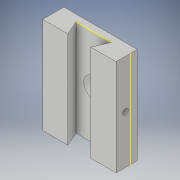
# Autodesk Inventor part: 7.1 Schlitten
Saved by Autodesk Inventor 2018.3 (Build 223284000, 284)
## iProperties
Created: 2018-10-11
Part Number: 7.1 Schlitten
Material: Generisch
Document SubType Name: Modeling
Designer: pgmadmin
Density: 1 g/cm^3
Appearance: Vorgabe
Author: pgmadmin
Autodesk Inventor part; units mm, degrees
ref_plane "YZ Plane" through (0, 0, 0) normal (1, 0, 0) x (0, 1, 0)
ref_plane "XZ Plane" through (0, 0, 0) normal (0, 1, 0) x (-1, 0, 0)
ref_plane "XY Plane" through (0, 0, 0) normal (0, 0, 1) x (1, 0, 0)
sketch "Skizze1" plane through (0, 0, 0) normal (0, 0, 1) x (1, 0, 0)
  line L0 (-18.1618, 0.375) -> (-21.3761, 7.875)
  line L1 (-2.9476, 7.875) -> (-6.1618, 0.375)
  line L2 (-6.1618, 0.375) -> (-18.1618, 0.375)
  line L3 (-18.1618, 0.375) -> (-31.1618, 0.375)
  line L4 (-31.1618, 0.375) -> (-31.1618, 11.375)
  line L5 (-31.1618, 11.375) -> (6.8382, 11.375)
  line L6 (6.8382, 11.375) -> (6.8382, 0.375)
  line L7 (6.8382, 0.375) -> (-6.1618, 0.375)
  line L8 (-21.5376, 7.875) -> (-2.9476, 7.875)
  point P0 (0, 0)
  point P1 (-21.1618, 7.375)
  point P2 (-3.1618, 7.375)
  dimension "d10" = 38
  dimension "d14" = 12
  dimension "d29" = 13
  constraints: 18 end point, 4 perpendicular, 4 point on line, 2 horizontal, 1 collinear
  measures "d10" distance of L4.end L5.end
  measures "d14" distance of L1.end L0.start
  measures "d29" distance of L0.start L3.end
extrude "Extrusion1" add sketch "Skizze1" along normal blind 50 contours L3 L4 L5 L6 L7 L1 L8 L0
sketch "Skizze2" plane through (6.8382, 0.375, 0) normal (1, 0, 0) x (0, 0, -1)
  line L0 (-50, 0) -> (-50, 11) projected
  line L1 (0, 11) -> (-50, 11) projected
  point P0 (0, -0.375)
  point P1 (-25, 4.85)
  dimension "d19" = 6.15
  measures "d19" distance from line of L1 point (-25, 4.85)
hole "Bohrung1" at (6.8382, 5.225, 25) direction (-1, 0, 0) diameter 2.9 depth 8 tip angle 118
sketch "Skizze3" plane through (-21.3761, 7.875, 0) normal (0, -1, 0) x (1, 0, 0)
  line L0 (0, 50) -> (18.4286, 50) projected
  line L1 (28.2143, 0) -> (28.2143, 50) projected
  point P0 (21.3761, 0)
sketch "Skizze4" plane through (-21.3761, 7.875, 0) normal (0, -1, 0) x (1, 0, 0)
  line L0 (0, 50) -> (18.4286, 50) projected
  line L1 (28.2143, 0) -> (28.2143, 50) projected
  point P0 (21.3761, 0)
  point P1 (9.2143, 25)
  dimension "d30" = 25
  dimension "d31" = 19
  measures "d30" distance from line of L0 point (9.214, 25)
  measures "d31" distance from line of L1 point (9.214, 25)
hole "Bohrung2" at (-12.1618, 7.875, 25) direction (0, 1, 0) diameter 5.2 end through all countersink diameter 10.5 countersink angle 90
sketch "Skizze5" plane through (-31.1618, 11.375, 0) normal (0, 1, 0) x (1, 0, 0)
  line L0 (0, 0) -> (0, -50) projected
  line L1 (38, 0) -> (38, -50) projected
  line L2 (38, -49) -> (0, -49)
  line L3 (0, -1) -> (38, -1)
  line L4 (38, 0) -> (0, 0) projected
  line L5 (38, -50) -> (0, -50) projected
  line L6 (24.3865, -1) -> (24.8517, -1)
  line L7 (24.8517, -1) -> (24.8517, -2.7131)
  line L8 (24.8517, -2.7131) -> (26.4627, -2.7131)
  line L9 (26.4627, -2.7131) -> (26.4627, -1)
  line L10 (26.4627, -1) -> (26.9279, -1)
  line L11 (26.9279, -1) -> (26.9279, -4.5)
  line L12 (26.9279, -4.5) -> (26.4627, -4.5)
  line L13 (26.4627, -4.5) -> (26.4627, -3.1272)
  line L14 (26.4627, -3.1272) -> (24.8517, -3.1272)
  line L15 (24.8517, -3.1272) -> (24.8517, -4.5)
  line L16 (24.8517, -4.5) -> (24.3865, -4.5)
  line L17 (24.3865, -4.5) -> (24.3865, -1)
  spline S0 degree 2 poles (21.5531, -2.3132) (21.5531, -1.6495) (22.1912, -0.9263) (22.7245, -0.9263) knots 0 0 0 1 2 2 2
  spline S1 degree 2 poles (22.7245, -0.9263) (23.2719, -0.9263) (23.8987, -1.6722) (23.8987, -2.3132) knots 0 0 0 1 2 2 2
  spline S2 degree 2 poles (23.8987, -2.3132) (23.8987, -2.9712) (23.252, -3.7002) (22.7245, -3.7002) knots 0 0 0 1 2 2 2
  spline S3 degree 2 poles (22.7245, -3.7002) (22.1912, -3.7002) (21.5531, -2.9741) (21.5531, -2.3132) knots 0 0 0 1 2 2 2
  spline S4 degree 2 poles (22.0097, -2.3132) (22.0097, -2.8237) (22.3813, -3.3201) (22.7245, -3.3201) knots 0 0 0 1 2 2 2
  spline S5 degree 2 poles (22.7245, -3.3201) (23.0677, -3.3201) (23.4421, -2.8237) (23.4421, -2.3132) knots 0 0 0 1 2 2 2
  spline S6 degree 2 poles (23.4421, -2.3132) (23.4421, -1.8169) (23.0677, -1.3063) (22.7245, -1.3063) knots 0 0 0 1 2 2 2
  spline S7 degree 2 poles (22.7245, -1.3063) (22.3841, -1.3063) (22.0097, -1.8083) (22.0097, -2.3132) knots 0 0 0 1 2 2 2
  line L18 (20.6483, -1) -> (21.0908, -1)
  line L19 (21.0908, -1) -> (21.0908, -4.656)
  line L20 (21.0908, -4.656) -> (20.6483, -4.656)
  line L21 (20.6483, -4.656) -> (20.6483, -1)
  line L22 (16.9639, -1) -> (17.4291, -1)
  line L23 (17.4291, -1) -> (17.4291, -4.015)
  line L24 (17.4291, -4.015) -> (18.3424, -1.9643)
  line L25 (18.3424, -1.9643) -> (18.626, -1.9643)
  line L26 (18.626, -1.9643) -> (19.5308, -4.015)
  line L27 (19.5308, -4.015) -> (19.5308, -1)
  line L28 (19.5308, -1) -> (19.9648, -1)
  line L29 (19.9648, -1) -> (19.9648, -4.5)
  line L30 (19.9648, -4.5) -> (19.3294, -4.5)
  line L31 (19.3294, -4.5) -> (18.4558, -2.5515)
  line L32 (18.4558, -2.5515) -> (17.6106, -4.5)
  line L33 (17.6106, -4.5) -> (16.9639, -4.5)
  line L34 (16.9639, -4.5) -> (16.9639, -1)
  spline S8 degree 2 poles (13.7788, -4.1001) (13.5802, -3.8675) (13.359, -3.1868) (13.359, -2.75) knots 0 0 0 1 2 2 2
  spline S9 degree 2 poles (13.359, -2.75) (13.359, -2.3246) (13.5746, -1.6353) (13.7788, -1.4028) knots 0 0 0 1 2 2 2
  spline S10 degree 2 poles (13.7788, -1.4028) (13.9943, -1.1588) (14.5644, -0.9263) (14.9076, -0.9263) knots 0 0 0 1 2 2 2
  spline S11 degree 2 poles (14.9076, -0.9263) (15.2622, -0.9263) (15.8294, -1.1673) (16.0365, -1.4028) knots 0 0 0 1 2 2 2
  spline S12 degree 2 poles (16.0365, -1.4028) (16.2378, -1.6353) (16.4534, -2.3189) (16.4534, -2.75) knots 0 0 0 1 2 2 2
  spline S13 degree 2 poles (16.4534, -2.75) (16.4534, -3.1896) (16.235, -3.859) (16.0336, -4.1001) knots 0 0 0 1 2 2 2
  spline S14 degree 2 poles (16.0336, -4.1001) (15.8294, -4.3327) (15.2593, -4.5737) (14.9076, -4.5737) knots 0 0 0 1 2 2 2
  spline S15 degree 2 poles (14.9076, -4.5737) (14.5502, -4.5737) (13.9773, -4.3241) (13.7788, -4.1001) knots 0 0 0 1 2 2 2
  spline S16 degree 2 poles (13.844, -2.75) (13.844, -3.096) (13.9943, -3.6321) (14.1305, -3.8079) knots 0 0 0 1 2 2 2
  spline S17 degree 2 poles (14.1305, -3.8079) (14.2695, -3.9895) (14.6609, -4.171) (14.9048, -4.171) knots 0 0 0 1 2 2 2
  spline S18 degree 2 poles (14.9048, -4.171) (15.1572, -4.171) (15.5373, -3.9951) (15.6819, -3.8079) knots 0 0 0 1 2 2 2
  spline S19 degree 2 poles (15.6819, -3.8079) (15.8209, -3.6293) (15.9684, -3.0904) (15.9684, -2.75) knots 0 0 0 1 2 2 2
  spline S20 degree 2 poles (15.9684, -2.75) (15.9684, -2.0608) (15.3898, -1.329) (14.9048, -1.329) knots 0 0 0 1 2 2 2
  spline S21 degree 2 poles (14.9048, -1.329) (14.4198, -1.329) (13.844, -2.0608) (13.844, -2.75) knots 0 0 0 1 2 2 2
  spline S22 degree 2 poles (11.8728, -0.9376) (12.2528, -0.9376) (12.7861, -1.0964) (13.0215, -1.2099) knots 0 0 0 1 2 2 2
  line L35 (13.0215, -1.2099) -> (13.0215, -1.7942)
  line L36 (13.0215, -1.7942) -> (12.9874, -1.7942)
  spline S23 degree 2 poles (12.9874, -1.7942) (12.7577, -1.5786) (12.1763, -1.3404) (11.9068, -1.3404) knots 0 0 0 1 2 2 2
  spline S24 degree 2 poles (11.9068, -1.3404) (11.5211, -1.3404) (11.1268, -1.6609) (11.1268, -1.9246) knots 0 0 0 1 2 2 2
  spline S25 degree 2 poles (11.1268, -1.9246) (11.1268, -2.1345) (11.3339, -2.3955) (11.5579, -2.4607) knots 0 0 0 1 2 2 2
  spline S26 degree 2 poles (11.5579, -2.4607) (11.7196, -2.5061) (11.9891, -2.5685) (12.1904, -2.6195) knots 0 0 0 1 2 2 2
  spline S27 degree 2 poles (12.1904, -2.6195) (12.372, -2.6677) (12.6584, -2.8124) (12.769, -2.9287) knots 0 0 0 1 2 2 2
  spline S28 degree 2 poles (12.769, -2.9287) (12.8768, -3.045) (12.9959, -3.357) (12.9959, -3.5612) knots 0 0 0 1 2 2 2
  spline S29 degree 2 poles (12.9959, -3.5612) (12.9959, -3.9866) (12.3323, -4.5624) (11.8189, -4.5624) knots 0 0 0 1 2 2 2
  spline S30 degree 2 poles (11.8189, -4.5624) (11.5239, -4.5624) (11.002, -4.4461) (10.778, -4.3355) knots 0 0 0 1 2 2 2
  line L37 (10.778, -4.3355) -> (10.778, -3.7796)
  line L38 (10.778, -3.7796) -> (10.812, -3.7796)
  spline S31 degree 2 poles (10.812, -3.7796) (10.9793, -3.9327) (11.5012, -4.1596) (11.7877, -4.1596) knots 0 0 0 1 2 2 2
  spline S32 degree 2 poles (11.7877, -4.1596) (12.111, -4.1596) (12.5109, -3.8562) (12.5109, -3.6094) knots 0 0 0 1 2 2 2
  spline S33 degree 2 poles (12.5109, -3.6094) (12.5109, -3.3882) (12.2755, -3.1244) (12.0543, -3.0648) knots 0 0 0 1 2 2 2
  spline S34 degree 2 poles (12.0543, -3.0648) (11.9068, -3.0251) (11.4785, -2.923) (11.3367, -2.8805) knots 0 0 0 1 2 2 2
  spline S35 degree 2 poles (11.3367, -2.8805) (10.9765, -2.7699) (10.6418, -2.3246) (10.6418, -1.9984) knots 0 0 0 1 2 2 2
  spline S36 degree 2 poles (10.6418, -1.9984) (10.6418, -1.7913) (10.8092, -1.3942) (10.9595, -1.2553) knots 0 0 0 1 2 2 2
  spline S37 degree 2 poles (10.9595, -1.2553) (11.1268, -1.1021) (11.5523, -0.9376) (11.8728, -0.9376) knots 0 0 0 1 2 2 2
  line L39 (13.4186, -49) -> (12.9534, -49)
  line L40 (12.9534, -49) -> (12.9534, -47.2869)
  line L41 (12.9534, -47.2869) -> (11.3424, -47.2869)
  line L42 (11.3424, -47.2869) -> (11.3424, -49)
  line L43 (11.3424, -49) -> (10.8772, -49)
  line L44 (10.8772, -49) -> (10.8772, -45.5)
  line L45 (10.8772, -45.5) -> (11.3424, -45.5)
  line L46 (11.3424, -45.5) -> (11.3424, -46.8728)
  line L47 (11.3424, -46.8728) -> (12.9534, -46.8728)
  line L48 (12.9534, -46.8728) -> (12.9534, -45.5)
  line L49 (12.9534, -45.5) -> (13.4186, -45.5)
  line L50 (13.4186, -45.5) -> (13.4186, -49)
  spline S38 degree 2 poles (16.252, -47.6868) (16.252, -48.3505) (15.6139, -49.0737) (15.0806, -49.0737) knots 0 0 0 1 2 2 2
  spline S39 degree 2 poles (15.0806, -49.0737) (14.5332, -49.0737) (13.9064, -48.3278) (13.9064, -47.6868) knots 0 0 0 1 2 2 2
  spline S40 degree 2 poles (13.9064, -47.6868) (13.9064, -47.0288) (14.5531, -46.2998) (15.0806, -46.2998) knots 0 0 0 1 2 2 2
  spline S41 degree 2 poles (15.0806, -46.2998) (15.6139, -46.2998) (16.252, -47.0259) (16.252, -47.6868) knots 0 0 0 1 2 2 2
  spline S42 degree 2 poles (15.7954, -47.6868) (15.7954, -47.1763) (15.4238, -46.6799) (15.0806, -46.6799) knots 0 0 0 1 2 2 2
  spline S43 degree 2 poles (15.0806, -46.6799) (14.7374, -46.6799) (14.363, -47.1763) (14.363, -47.6868) knots 0 0 0 1 2 2 2
  spline S44 degree 2 poles (14.363, -47.6868) (14.363, -48.1831) (14.7374, -48.6937) (15.0806, -48.6937) knots 0 0 0 1 2 2 2
  spline S45 degree 2 poles (15.0806, -48.6937) (15.421, -48.6937) (15.7954, -48.1917) (15.7954, -47.6868) knots 0 0 0 1 2 2 2
  line L51 (17.1568, -49) -> (16.7143, -49)
  line L52 (16.7143, -49) -> (16.7143, -45.344)
  line L53 (16.7143, -45.344) -> (17.1568, -45.344)
  line L54 (17.1568, -45.344) -> (17.1568, -49)
  line L55 (20.8412, -49) -> (20.376, -49)
  line L56 (20.376, -49) -> (20.376, -45.985)
  line L57 (20.376, -45.985) -> (19.4627, -48.0357)
  line L58 (19.4627, -48.0357) -> (19.1791, -48.0357)
  line L59 (19.1791, -48.0357) -> (18.2743, -45.985)
  line L60 (18.2743, -45.985) -> (18.2743, -49)
  line L61 (18.2743, -49) -> (17.8404, -49)
  line L62 (17.8404, -49) -> (17.8404, -45.5)
  line L63 (17.8404, -45.5) -> (18.4757, -45.5)
  line L64 (18.4757, -45.5) -> (19.3493, -47.4485)
  line L65 (19.3493, -47.4485) -> (20.1945, -45.5)
  line L66 (20.1945, -45.5) -> (20.8412, -45.5)
  line L67 (20.8412, -45.5) -> (20.8412, -49)
  spline S46 degree 2 poles (24.0263, -45.8999) (24.2249, -46.1325) (24.4461, -46.8132) (24.4461, -47.25) knots 0 0 0 1 2 2 2
  spline S47 degree 2 poles (24.4461, -47.25) (24.4461, -47.6754) (24.2306, -48.3647) (24.0263, -48.5972) knots 0 0 0 1 2 2 2
  spline S48 degree 2 poles (24.0263, -48.5972) (23.8108, -48.8412) (23.2407, -49.0737) (22.8975, -49.0737) knots 0 0 0 1 2 2 2
  spline S49 degree 2 poles (22.8975, -49.0737) (22.543, -49.0737) (21.9757, -48.8327) (21.7686, -48.5972) knots 0 0 0 1 2 2 2
  spline S50 degree 2 poles (21.7686, -48.5972) (21.5673, -48.3647) (21.3517, -47.6811) (21.3517, -47.25) knots 0 0 0 1 2 2 2
  spline S51 degree 2 poles (21.3517, -47.25) (21.3517, -46.8104) (21.5701, -46.141) (21.7715, -45.8999) knots 0 0 0 1 2 2 2
  spline S52 degree 2 poles (21.7715, -45.8999) (21.9757, -45.6673) (22.5458, -45.4263) (22.8975, -45.4263) knots 0 0 0 1 2 2 2
  spline S53 degree 2 poles (22.8975, -45.4263) (23.2549, -45.4263) (23.8278, -45.6759) (24.0263, -45.8999) knots 0 0 0 1 2 2 2
  spline S54 degree 2 poles (23.9611, -47.25) (23.9611, -46.904) (23.8108, -46.3679) (23.6746, -46.1921) knots 0 0 0 1 2 2 2
  spline S55 degree 2 poles (23.6746, -46.1921) (23.5357, -46.0105) (23.1442, -45.829) (22.9003, -45.829) knots 0 0 0 1 2 2 2
  spline S56 degree 2 poles (22.9003, -45.829) (22.6479, -45.829) (22.2678, -46.0049) (22.1232, -46.1921) knots 0 0 0 1 2 2 2
  spline S57 degree 2 poles (22.1232, -46.1921) (21.9842, -46.3707) (21.8367, -46.9096) (21.8367, -47.25) knots 0 0 0 1 2 2 2
  spline S58 degree 2 poles (21.8367, -47.25) (21.8367, -47.9392) (22.4153, -48.671) (22.9003, -48.671) knots 0 0 0 1 2 2 2
  spline S59 degree 2 poles (22.9003, -48.671) (23.3853, -48.671) (23.9611, -47.9392) (23.9611, -47.25) knots 0 0 0 1 2 2 2
  spline S60 degree 2 poles (25.9323, -49.0624) (25.5523, -49.0624) (25.019, -48.9036) (24.7836, -48.7901) knots 0 0 0 1 2 2 2
  line L68 (24.7836, -48.7901) -> (24.7836, -48.2058)
  line L69 (24.7836, -48.2058) -> (24.8177, -48.2058)
  spline S61 degree 2 poles (24.8177, -48.2058) (25.0474, -48.4214) (25.6288, -48.6596) (25.8983, -48.6596) knots 0 0 0 1 2 2 2
  spline S62 degree 2 poles (25.8983, -48.6596) (26.284, -48.6596) (26.6783, -48.3391) (26.6783, -48.0754) knots 0 0 0 1 2 2 2
  spline S63 degree 2 poles (26.6783, -48.0754) (26.6783, -47.8655) (26.4712, -47.6045) (26.2472, -47.5393) knots 0 0 0 1 2 2 2
  spline S64 degree 2 poles (26.2472, -47.5393) (26.0855, -47.4939) (25.816, -47.4315) (25.6147, -47.3805) knots 0 0 0 1 2 2 2
  spline S65 degree 2 poles (25.6147, -47.3805) (25.4331, -47.3323) (25.1467, -47.1876) (25.0361, -47.0713) knots 0 0 0 1 2 2 2
  spline S66 degree 2 poles (25.0361, -47.0713) (24.9283, -46.955) (24.8092, -46.643) (24.8092, -46.4388) knots 0 0 0 1 2 2 2
  spline S67 degree 2 poles (24.8092, -46.4388) (24.8092, -46.0134) (25.4729, -45.4376) (25.9862, -45.4376) knots 0 0 0 1 2 2 2
  spline S68 degree 2 poles (25.9862, -45.4376) (26.2812, -45.4376) (26.8031, -45.5539) (27.0271, -45.6645) knots 0 0 0 1 2 2 2
  line L70 (27.0271, -45.6645) -> (27.0271, -46.2204)
  line L71 (27.0271, -46.2204) -> (26.9931, -46.2204)
  spline S69 degree 2 poles (26.9931, -46.2204) (26.8258, -46.0673) (26.3039, -45.8404) (26.0174, -45.8404) knots 0 0 0 1 2 2 2
  spline S70 degree 2 poles (26.0174, -45.8404) (25.6941, -45.8404) (25.2942, -46.1438) (25.2942, -46.3906) knots 0 0 0 1 2 2 2
  spline S71 degree 2 poles (25.2942, -46.3906) (25.2942, -46.6118) (25.5296, -46.8756) (25.7508, -46.9352) knots 0 0 0 1 2 2 2
  spline S72 degree 2 poles (25.7508, -46.9352) (25.8983, -46.9749) (26.3266, -47.077) (26.4684, -47.1195) knots 0 0 0 1 2 2 2
  spline S73 degree 2 poles (26.4684, -47.1195) (26.8286, -47.2301) (27.1633, -47.6754) (27.1633, -48.0016) knots 0 0 0 1 2 2 2
  spline S74 degree 2 poles (27.1633, -48.0016) (27.1633, -48.2087) (26.9959, -48.6058) (26.8456, -48.7447) knots 0 0 0 1 2 2 2
  spline S75 degree 2 poles (26.8456, -48.7447) (26.6783, -48.8979) (26.2528, -49.0624) (25.9323, -49.0624) knots 0 0 0 1 2 2 2
  point P0 (31.1618, 0)
  dimension "d39" = 1
  dimension "d40" = 1
  constraints: 4 end point, 4 horizontal, 3 point on line
  measures "d39" distance between parallel lines of L4 L3
  measures "d40" distance between parallel lines of L5 L2
extrude "Extrusion2" cut sketch "Skizze5" against normal blind 2 contours S37 S22 L3 | L3 S22 L35 L36 S23 S24 S25 S26 S27 S28 S29 S30 L37 L38 S31 S32 S33 S34 S35 S36 S37 | L44 L45 L46 L47 L48 L49 L50 L2 L40 L41 L42 | L11 L12 L13 L14 L15 L16 L17 L3 L7 L8 L9 | S10 S11 L3 | L3 S11 S12 S13 S14 S15 S8 S9 S10 | S75 S60 L2 | L2 S60 L68 L69 S61 S62 S63 S64 S65 S66 S67 S68 L70 L71 S69 S70 S71 S72 S73 S74 S75 | L3 L23 L24 L25 L26 L27 L29 L30 L31 L32 L33 L34 | S48 S49 L2 | L2 S49 S50 S51 S52 S53 S46 S47 S48 | S39 S40 S41 S38 L2 | L2 S38 S39 | S1 S2 S3 S0 L3 | L3 S0 S1 | L2 L56 L57 L58 L59 L60 L62 L63 L64 L65 L66 L67 | L52 L53 L54 L2 | L19 L20 L21 L3
